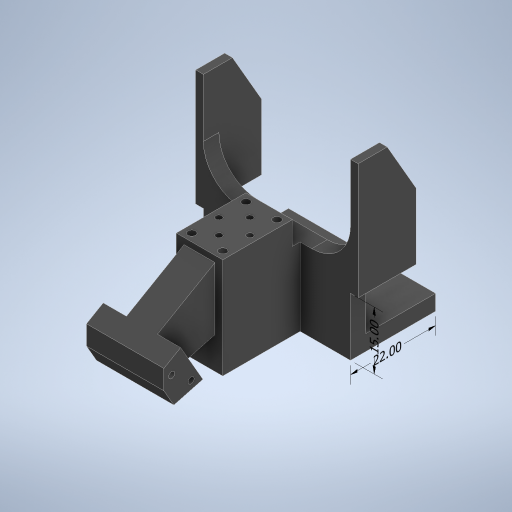
# Autodesk Inventor part: hipjoint_middle
Saved by Autodesk Inventor 2024.1 (Build 281209000, 209)
## iProperties
Created: 2024-10-09
Part Number: hipjoint_middle
Material: 一般
Document SubType Name: Modeling
Designer: hibik
Density: 1 g/cm^3
Appearance: 既定
Author: hibik
Autodesk Inventor part; units mm, degrees
ref_plane "YZ Plane" through (0, 0, 0) normal (1, 0, 0) x (0, 1, 0)
ref_plane "XZ Plane" through (0, 0, 0) normal (0, 1, 0) x (-1, 0, 0)
ref_plane "XY Plane" through (0, 0, 0) normal (0, 0, 1) x (1, 0, 0)
sketch "スケッチ1" plane through (0, 0, 0) normal (0, 1, 0) x (-1, 0, 0)
  line L0 (-6, -13) -> (6, -13)
  line L1 (6, -13) -> (6, 13)
  line L2 (6, 13) -> (-6, 13)
  line L3 (-6, 13) -> (-6, -13)
  line L4 (-6, -13) -> (6, 13) construction
  line L5 (6, -13) -> (-6, 13) construction
  line L6 (6, 13) -> (-6, 13)
  line L7 (-6, 13) -> (-6, 5)
  line L8 (-6, 5) -> (6, 5)
  line L9 (6, 5) -> (6, 13)
  point P0 (0, 0)
  point P1 (0, 13)
  point P2 (-6, 13)
  point P3 (6, 5)
  dimension "d0" = 12
  dimension "d1" = 26
  dimension "d26" = 12
  dimension "d27" = 8
  constraints: 20 end point, 4 midpoint, 4 parallel, 2 horizontal, 2 perpendicular, 1 point on line
  measures "d0" distance of L2.end L1.end
  measures "d1" distance of L1.end L0.end
  measures "d26" distance of L8.end L7.end
  measures "d27" distance of L7.end L6.end
extrude "押し出し1" add sketch "スケッチ1" against normal blind 3 contours L3 L8 L1 L0
sketch "スケッチ5" plane through (0, 0, 0) normal (1, 0, 0) x (0, 1, 0)
  line L0 (-3, 5) -> (-3, -13) projected
  line L1 (-3, 5) -> (-3, 13)
  line L2 (-1.6051, 5) -> (-12.6984, 24.2141)
  line L3 (-12.6984, 24.2141) -> (-17.6984, 24.2141)
  line L4 (-16.3866, 0) -> (-3, 0)
  line L5 (0, 5) -> (-3, 5) projected
  line L6 (-17.6984, 24.2141) -> (-22.1813, 21.6259)
  line L7 (-22.1813, 21.6259) -> (-16.3866, 0)
  line L8 (-12.6984, 24.2141) -> (-8.3683, 26.7141) construction
  line L9 (-8.3683, 26.7141) -> (-7.6183, 25.4151) construction
  circle A0 centre (-7.6183, 25.4151) radius 1 construction
  line L10 (36.5, 48) -> (-6.3683, 23.25) construction
  line L11 (0, 13) -> (36.5, 13) construction
  line L12 (0, -13) -> (0, 5) projected
  line L13 (-3, 5) -> (-1.6051, 5)
  point P0 (0, 0)
  dimension "d28" = 8
  dimension "d29" = 120
  dimension "d31" = 5
  dimension "d32" = 5
  dimension "d35" = 5
  dimension "d36" = 150
  dimension "d37" = 75
  dimension "d47" = 5
  dimension "d48" = 1.5
  dimension "d49" = 2
  dimension "d50" = 2.5
  dimension "d51" = 49.5
  dimension "d53" = 8
  dimension "d54" = 36.5
  dimension "d55" = 35
  constraints: 22 end point, 5 perpendicular, 3 horizontal, 2 point on line, 2 vertical alignment, 1 centre point, 1 coincident, 1 vertical
  measures "d28" distance of L0.start L1.end
  measures "d29" angle of L5 L2
  measures "d31" distance between parallel lines of L4 L5
  measures "d32" distance of L2.end L3.end
  measures "d35" distance from line of L3.end L7
  measures "d36" angle of L3 L6
  measures "d37" angle of L6 L7
  measures "d47" distance from line of L8.end L2
  measures "d48" distance of L8.end L9.end
  measures "d49" diameter of A0
  measures "d50" distance from line of L9.end L10
  measures "d51" distance from line of L10.start L9
  measures "d53" distance from line of L11 L5.start
  measures "d54" distance of L11.start L11.end
  measures "d55" distance from line of L10.start L11
extrude "押し出し5" add sketch "スケッチ5" against normal blind 4
sketch "スケッチ6" plane through (-4, 0, 0) normal (-1, 0, 0) x (0, 0, 1)
  line L0 (0, -3) -> (0, -16.3866) projected
  line L1 (0, -16.3866) -> (21.6259, -22.1813) projected
  line L2 (21.6259, -22.1813) -> (24.2141, -17.6984) projected
  line L3 (24.2141, -17.6984) -> (24.2141, -12.6984) projected
  line L4 (24.2141, -12.6984) -> (5, -1.6051) projected
  line L5 (0, -3) -> (5, -3) projected
  line L6 (19.884, -10.1984) -> (14.1259, -20.1716)
  line L7 (24.2141, -12.6984) -> (5.604, -1.9538) projected
  line L8 (5, -3) -> (5, -1.6051) projected
  point P0 (0, 0)
  dimension "d38" = 5
  constraints: 2 end point, 2 point on line, 2 other
  measures "d38" distance from line of L3.end L6
extrude "押し出し6" add sketch "スケッチ6" along normal blind 6 contours L6 L4 L3 L2 L1
mirror "ミラー3" about plane through (0, -11.8932, 12.1071) normal (1, 0, 0) of "押し出し5", "押し出し6"
sketch "スケッチ7" plane through (0, 0, 0) normal (0, 1, 0) x (1, 0, 0)
  circle A0 centre (4, -3) radius 1 projected
  circle A1 centre (-4, 11) radius 1 projected
  circle A2 centre (0, 0) radius 0.8 projected
  circle A3 centre (0, 8) radius 0.8 projected
  circle A4 centre (-4, 4) radius 0.8 projected
  circle A5 centre (4, 4) radius 0.8 projected
  circle A6 centre (4, 11) radius 1 projected
  circle A7 centre (-4, -3) radius 1 projected
  line L0 (6, -8) -> (6, -10) projected
  line L1 (30, -13) -> (9, -13) projected
  line L2 (33, -9.25) -> (33, -10) projected
  arc A8 (30, 6.25) -> (30, -6.25) centre (30, 0) ccw projected
  line L3 (33, 10) -> (33, 9.25) projected
  line L4 (-30, 13) -> (30, 13) projected
  line L5 (-33, -10) -> (-33, -9.25) projected
  arc A9 (-30, -6.25) -> (-30, 6.25) centre (-30, 0) ccw projected
  line L6 (-33, 9.25) -> (-33, 10) projected
  line L7 (-9, -13) -> (-30, -13) projected
  line L8 (-6, -10) -> (-6, -8) projected
  line L9 (-3, -5) -> (3, -5) projected
  line L10 (21.75, 7.5) -> (21.75, -7.5) projected
  line L11 (18.75, -10.5) -> (14, -10.5) projected
  line L12 (11, -7.5) -> (11, 7.5) projected
  line L13 (14, 10.5) -> (18.75, 10.5) projected
  circle A10 centre (9, 10.5) radius 0.85 projected
  circle A11 centre (30, -10.5) radius 0.85 projected
  circle A12 centre (-30, -10.5) radius 0.85 projected
  circle A13 centre (-9, 10.5) radius 0.85 projected
  circle A14 centre (-30, 10.5) radius 0.85 projected
  circle A15 centre (-9, -10.5) radius 0.85 projected
  circle A16 centre (9, -10.5) radius 0.85 projected
  circle A17 centre (30, 10.5) radius 0.85 projected
  line L14 (-11, 7.5) -> (-11, -7.5) projected
  line L15 (-14, -10.5) -> (-18.75, -10.5) projected
  line L16 (-21.75, -7.5) -> (-21.75, 7.5) projected
  line L17 (-18.75, 10.5) -> (-14, 10.5) projected
  arc A18 (-30, 13) -> (-33, 10) centre (-30, 10) ccw projected
  arc A19 (-33, 9.25) -> (-30, 6.25) centre (-30, 9.25) ccw projected
  arc A20 (-30, -6.25) -> (-33, -9.25) centre (-30, -9.25) ccw projected
  arc A21 (-33, -10) -> (-30, -13) centre (-30, -10) ccw projected
  arc A22 (-9, -13) -> (-6, -10) centre (-9, -10) ccw projected
  arc A23 (-3, -5) -> (-6, -8) centre (-3, -8) ccw projected
  arc A24 (6, -8) -> (3, -5) centre (3, -8) ccw projected
  arc A25 (6, -10) -> (9, -13) centre (9, -10) ccw projected
  arc A26 (30, -13) -> (33, -10) centre (30, -10) ccw projected
  arc A27 (33, -9.25) -> (30, -6.25) centre (30, -9.25) ccw projected
  arc A28 (30, 6.25) -> (33, 9.25) centre (30, 9.25) ccw projected
  arc A29 (33, 10) -> (30, 13) centre (30, 10) ccw projected
  arc A30 (-14, -10.5) -> (-11, -7.5) centre (-14, -7.5) ccw projected
  arc A31 (-21.75, -7.5) -> (-18.75, -10.5) centre (-18.75, -7.5) ccw projected
  arc A32 (-18.75, 10.5) -> (-21.75, 7.5) centre (-18.75, 7.5) ccw projected
  arc A33 (-11, 7.5) -> (-14, 10.5) centre (-14, 7.5) ccw projected
  arc A34 (18.75, -10.5) -> (21.75, -7.5) centre (18.75, -7.5) ccw projected
  arc A35 (11, -7.5) -> (14, -10.5) centre (14, -7.5) ccw projected
  arc A36 (14, 10.5) -> (11, 7.5) centre (14, 7.5) ccw projected
  arc A37 (21.75, 7.5) -> (18.75, 10.5) centre (18.75, 7.5) ccw projected
  point P0 (0, 0)
extrude "押し出し7" cut sketch "スケッチ7" against normal up to surface (3 mm away) contours A0 | A1 | A2 | A3 | A4 | A5 | A6 | A7
sketch "スケッチ8" plane through (0, -3, 0) normal (0, -1, 0) x (1, 0, 0)
  line L0 (-6, 5) -> (6, 5) projected
  line L1 (-6, -13) -> (-6, 5) projected
  line L2 (6, -13) -> (-6, -13) projected
  line L3 (6, 5) -> (6, -13) projected
  point P0 (0, 0)
extrude "押し出し8" add sketch "スケッチ8" along normal blind 23
sketch "スケッチ9" plane through (0, -26, 0) normal (0, -1, 0) x (1, 0, 0)
  circle A0 centre (-4, 3) radius 1 projected
  circle A1 centre (4, 3) radius 1 projected
  circle A2 centre (4, -11) radius 1 projected
  circle A3 centre (4, -11) radius 1 projected
  circle A4 centre (-4, -11) radius 1 projected
  circle A5 centre (-4, -11) radius 1 projected
  point P0 (0, 0)
extrude "押し出し9" cut sketch "スケッチ9" against normal blind 7
sketch "スケッチ10" plane through (10, -17.6984, 24.2141) normal (1, 0, 0) x (0, 0, -1)
  circle A0 centre (2, 2.5) radius 1 construction
  circle A1 centre (7.0529, -1.216) radius 1 construction
  circle A2 centre (2, 2.5) radius 0.8
  circle A3 centre (7.0529, -1.216) radius 0.8
  point P0 (24.2141, 17.6984)
  dimension "d56" = 1.6
  dimension "d57" = 1.6
  constraints: 2 centre point, 2 coincident
  measures "d56" diameter of A2
  measures "d57" diameter of A3
extrude "押し出し10" cut sketch "スケッチ10" against normal through all
sketch "スケッチ11" plane through (6, 0, 5) normal (1, 0, 0) x (0, 0, -1)
  line L0 (18, 0) -> (18, -26) projected
  line L1 (18, -11) -> (20, -11)
  line L2 (20, -11) -> (20, -26)
  line L3 (20, -26) -> (18, -26)
  line L4 (18, -26) -> (18, -11)
  line L5 (18, -26) -> (0, -26) projected
  point P0 (5, 0)
  dimension "d60" = 15
  dimension "d61" = 2
  constraints: 8 end point, 2 parallel, 1 collinear, 1 horizontal, 1 perpendicular, 1 point on line
  measures "d60" distance of L1.end L2.end
  measures "d61" distance of L2.end L3.end
extrude "押し出し11" add sketch "スケッチ11" against normal up to surface (12 mm away)
sketch "スケッチ12" plane through (0, 0, 0) normal (1, 0, 0) x (0, 1, 0)
  line L0 (-26, -15) -> (-11, -15) projected
  line L1 (-11, -15) -> (-26, -15)
  line L2 (-26, -15) -> (-26, -19)
  line L3 (-26, -19) -> (-11, -19)
  line L4 (-11, -19) -> (-11, -15)
  line L5 (-22, -19) -> (-26, -19)
  line L6 (-26, -19) -> (-26, -37)
  line L7 (-26, -37) -> (-22, -37)
  line L8 (-22, -37) -> (-22, -19)
  line L9 (-26, 5) -> (-26, -15) projected
  point P0 (0, 0)
  dimension "d64" = 4
  dimension "d65" = 4
  dimension "d66" = 18
  constraints: 16 end point, 4 parallel, 2 collinear, 2 horizontal, 2 perpendicular, 1 point on line
  measures "d64" distance of L2.end L1.end
  measures "d65" distance of L7.end L6.end
  measures "d66" distance of L7.end L5.start
extrude "押し出し12" add sketch "スケッチ12" against normal blind 19
mirror "ミラー4" about plane through (0, -18.5, -26) normal (1, 0, 0) of "押し出し12"
sketch "スケッチ13" plane through (-6, -11, -13) normal (0, 1, 0) x (1, 0, 0)
  line L0 (-15, 6) -> (27, 6)
  line L1 (27, 6) -> (27, 2)
  line L2 (27, 2) -> (-15, 2)
  line L3 (-15, 2) -> (-15, 6)
  line L4 (0, 2) -> (-13, 2) projected
  line L5 (-13, 6) -> (25, 6) projected
  line L6 (25, 2) -> (25, 6) projected
  line L7 (-15, 2) -> (-13, 2)
  line L8 (-13, 2) -> (-13, 17)
  line L9 (-13, 17) -> (-15, 17)
  line L10 (-15, 17) -> (-15, 2)
  line L11 (27, 2) -> (25, 2)
  line L12 (25, 2) -> (25, 17)
  line L13 (25, 17) -> (27, 17)
  line L14 (27, 17) -> (27, 2)
  line L15 (-13, 2) -> (-13, 6) projected
  point P0 (6, -13)
  point P1 (25, 6)
  point P2 (27, 6)
  point P3 (-13, 2)
  point P4 (-15, 6)
  dimension "d75" = 2
  dimension "d76" = 2
  dimension "d77" = 15
  constraints: 24 end point, 6 parallel, 5 collinear, 3 horizontal, 3 perpendicular
  measures "d75" distance from line of L3 L4.end
  measures "d76" distance between parallel lines of L6 L1
  measures "d77" distance of L9.end L2.end
extrude "押し出し13" add sketch "スケッチ13" along normal blind 30 contours L10 L9 L8 L0 | L0 L8 L2 L3 | L12 L13 L14 L0 | L0 L1 L2 L6
sketch "スケッチ14" plane through (-6, -11, -13) normal (0, 1, 0) x (1, 0, 0)
  line L0 (0, 2) -> (0, 0) projected
  line L1 (12, 0) -> (0, 0) projected
  line L2 (12, 2) -> (12, 0) projected
  line L3 (12, 2) -> (25, 2) projected
  line L4 (25, 2) -> (25, 6) projected
  line L5 (-13, 6) -> (25, 6) projected
  line L6 (-13, 2) -> (-13, 6) projected
  line L7 (0, 2) -> (-13, 2) projected
  point P0 (6, -13)
extrude "押し出し14" add sketch "スケッチ14" along normal blind 5
fillet "フィレット1" radius 10 2 edges at (-19, -6, -17) (19, -6, -17)
sketch "スケッチ16" plane through (21, -11, -15) normal (1, 0, 0) x (0, 0, -1)
  line L0 (15, 30) -> (0, 30) projected
  line L1 (7.5, 30) -> (15, 17.0096)
  line L2 (15, 0) -> (15, 30) projected
  point P0 (-15, 11)
  dimension "d85" = 120
  constraints: 2 end point, 1 midpoint, 1 point on line
  measures "d85" angle of L0 L1
extrude "押し出し16" cut sketch "スケッチ16" along normal through all both and the other way through all
equation "\"d76\" = d75"
